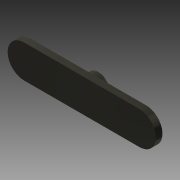
# Autodesk Inventor part: tang
Saved by Autodesk Inventor 2015 (Build 190159000, 159)
## iProperties
Created: 2015-06-11
Part Number: tang
Material: Generic
Document SubType Name: Modeling
Designer: david
Density: 1 g/cm^3
Appearance: Gunmetal
Mass: 0.893993 g
Surface Area: 11.8872 cm^2
Volume: 0.893993 cm^3
Author: david
Autodesk Inventor part; units mm, degrees
ref_plane "YZ Plane" through (0, 0, 0) normal (1, 0, 0) x (0, 1, 0)
ref_plane "XZ Plane" through (0, 0, 0) normal (0, 1, 0) x (-1, 0, 0)
ref_plane "XY Plane" through (0, 0, 0) normal (0, 0, 1) x (1, 0, 0)
sketch "Sketch1" plane through (0, 0, 0) normal (0, 1, 0) x (-1, 0, 0)
  line L0 (17.5, 0) -> (-17.5, 0) construction
  line L1 (17.5, 5) -> (-17.5, 5)
  line L2 (-17.5, -5) -> (17.5, -5)
  arc A0 (17.5, -5) -> (17.5, 5) centre (17.5, 0) ccw
  arc A1 (-17.5, 5) -> (-17.5, -5) centre (-17.5, 0) ccw
  point P0 (0, 0)
  dimension "d0" = 17.5
  dimension "d1" = 10
  constraints: 8 end point, 4 point on circle, 4 tangent, 2 centre point, 1 horizontal, 1 midpoint, 1 parallel
  measures "d0" distance of point (0, 0) L0.end
  measures "d1" diameter of A1
extrude "Extrusion1" add sketch "Sketch1" along normal blind 2
sketch "Sketch2" plane through (0, 2, 0) normal (0, 1, 0) x (1, 0, 0)
  circle A0 centre (0, 0) radius 3.5
  dimension "d4" = 7
  constraints: 1 centre point, 1 coincident
  measures "d4" diameter of A0
extrude "Extrusion2" add sketch "Sketch2" along normal blind 3
sketch "Sketch3" plane through (0, 5, 0) normal (0, 1, 0) x (1, 0, 0)
  circle A0 centre (0, 0) radius 2.5
  point P0 (0, 0)
  dimension "d7" = 5
  constraints: 1 centre point, 1 coincident
  measures "d7" diameter of A0
extrude "Extrusion3" cut sketch "Sketch3" against normal blind 4
body "Solid1"
